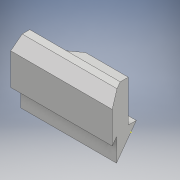
# Autodesk Inventor part: P3-14
Saved by Autodesk Inventor 2017 (Build 210142000, 142)
## iProperties
Created: 2017-02-13
Part Number: P3-14
Material: Generic
Document SubType Name: Modeling
Designer: Schaffel
Density: 1 g/cm^3
Appearance: Default
Author: Schaffel
Autodesk Inventor part; units mm, degrees
ref_plane "YZ Plane" through (0, 0, 0) normal (1, 0, 0) x (0, 1, 0)
ref_plane "XZ Plane" through (0, 0, 0) normal (0, 1, 0) x (-1, 0, 0)
ref_plane "XY Plane" through (0, 0, 0) normal (0, 0, 1) x (1, 0, 0)
sketch "Sketch1" plane through (0, 0, 0) normal (0, 0, 1) x (1, 0, 0)
  line L0 (0, 0) -> (80, 0)
  line L1 (80, 0) -> (144, 0) construction
  line L2 (80, 0) -> (54.0192, 45)
  line L3 (54.0192, 45) -> (29.0192, 45)
  line L4 (0, 0) -> (0, 15)
  line L5 (29.0192, 45) -> (29.0192, 15)
  line L6 (29.0192, 15) -> (0, 15)
  dimension "d0" = 80
  dimension "d2" = 25
  constraints: 14 end point, 3 horizontal, 2 vertical, 1 perpendicular
  measures "d0" distance of L0.start L0.end
  measures "d2" distance of L2.end L3.end
extrude "Extrusion1" add sketch "Sketch1" along normal blind 50
sketch "Sketch2" plane through (54.0192, 45, 50) normal (0.866, 0.5, 0) x (0, 0, -1)
  point P0 (50, -11.9615)
sketch "Sketch3" plane through (0, 0, 0) normal (-1, 0, 0) x (0, 0, 1)
  line L0 (50, 0) -> (50, 45) projected
  line L1 (50, 0) -> (50, 9)
  line L2 (50, 0) -> (43, 0)
  line L3 (0, 0) -> (50, 0) projected
  line L4 (43, 0) -> (50, 9)
  line L5 (0, 0) -> (18, 0)
  line L6 (0, 0) -> (0, 45) projected
  line L7 (0, 0) -> (0, 8)
  line L8 (18, 8) -> (18, 0)
  line L9 (18, 8) -> (0, 8)
  line L10 (0, 45) -> (0, 30)
  line L11 (0, 45) -> (20, 45) construction
  line L12 (0, 45) -> (8.6603, 30)
  line L13 (50, 15) -> (41.3397, 30)
  line L14 (41.3397, 30) -> (8.6603, 30)
  line L15 (0, 45) -> (50, 45) projected
  line L16 (0, 45) -> (50, 45)
  line L17 (50, 45) -> (50, 15)
  constraints: 28 end point, 6 point on line, 3 equal length, 2 horizontal, 2 perpendicular
extrude "Extrusion2" cut sketch "Sketch3" against normal blind 80 contours L2 L4 L0 | L13 L14 L12 L15 L0 | L3 L6 L9 L8
body "Solid1"
